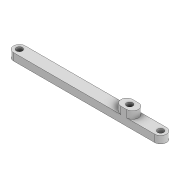
# Autodesk Inventor part: Part_7
Saved by Autodesk Inventor 2022 (Build 260153000, 153)
## iProperties
Created: 2022-04-21
Part Number: Part_7
Material: Generic
Document SubType Name: Modeling
Designer: dell
Density: 1 g/cm^3
Appearance: Default
Author: dell
Autodesk Inventor part; units mm, degrees
ref_plane "YZ Plane" through (0, 0, 0) normal (1, 0, 0) x (0, 1, 0)
ref_plane "XZ Plane" through (0, 0, 0) normal (0, 1, 0) x (-1, 0, 0)
ref_plane "XY Plane" through (0, 0, 0) normal (0, 0, 1) x (1, 0, 0)
sketch "Sketch1" plane through (0, 0, 0) normal (0, 1, 0) x (-1, 0, 0)
  line L0 (0, 0) -> (-96.842, 0) construction
  line L1 (0, 4) -> (-96.842, 4)
  line L2 (-96.842, -4) -> (0, -4)
  arc A0 (0, -4) -> (0, 4) centre (0, 0) ccw
  arc A1 (-96.842, 4) -> (-96.842, -4) centre (-96.842, 0) ccw
  circle A2 centre (0, 0) radius 2.1
  circle A3 centre (-96.842, 0) radius 2.1
  circle A4 centre (-75.611, 0) radius 2.1
  point P0 (-48.421, 0)
  dimension "d0" = 96.842
  dimension "d1" = 8
  dimension "d2" = 4.2
  dimension "d10" = 4.2
  dimension "d28" = 4.2
  dimension "d29" = 75.611
  constraints: 8 end point, 5 centre point, 4 point on circle, 4 tangent, 2 coincident, 1 horizontal, 1 midpoint, 1 parallel, 1 point on line
  measures "d0" distance of L0.end L0.start
  measures "d1" distance between parallel lines of L1 L2
  measures "d2" diameter of A2
  measures "d10" diameter of A3
  measures "d28" diameter of A4
  measures "d29" distance of L0.start A4.centre
extrude "Extrusion1" add sketch "Sketch1" along normal blind 5
sketch "Sketch4" plane through (0, 5, 0) normal (0, 1, 0) x (1, 0, 0)
  arc A0 (96.842, -4) -> (96.842, 4) centre (96.842, 0) ccw projected
  line L0 (96.842, 4) -> (0, 4) projected
  arc A1 (0, 4) -> (0, -4) centre (0, 0) ccw projected
  line L1 (0, -4) -> (96.842, -4) projected
  circle A2 centre (75.611, 0) radius 2.1 projected
  circle A3 centre (96.842, 0) radius 2.1 projected
  circle A4 centre (0, 0) radius 2.1 projected
  circle A5 centre (75.611, 0) radius 4
  circle A6 centre (73.611, 0) radius 4
  circle A7 centre (77.611, 0) radius 4
  point P0 (73.611, 4)
  point P1 (73.611, -4)
  point P2 (77.611, -4)
  point P3 (77.611, 4)
  dimension "d30" = 8
  dimension "d31" = 8
  dimension "d32" = 8
  dimension "d33" = 2
  dimension "d34" = 2
  constraints: 3 centre point, 1 coincident
  measures "d30" diameter of A5
  measures "d31" diameter of A6
  measures "d32" diameter of A7
  measures "d33" distance of A2.centre A6.centre
  measures "d34" distance of A7.centre A2.centre
extrude "Extrusion7" add sketch "Sketch4" along normal blind 5 contours L1 A5 A7 | A7 A5 | A7 A5 L0 | L1 A6 A5 | A5 A6 A7 | A7 A6 A2 A5 | A5 A6 L0 | A5 A7 A6 | A6 A5 | A5 A6 A7 A2 | A7 A2 A6 | A6 A2 A7 picked at (75.3898, -2.8494) picked at (75.3898, 2.8494)
body "Solid1"
